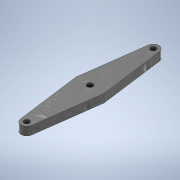
# Autodesk Inventor part: ServoXAxis
Saved by Autodesk Inventor 2022 (Build 260153000, 153)
## iProperties
Created: 2021-11-09
Part Number: ServoXAxis
Material: Generic
Document SubType Name: Modeling
Designer: Juan
Density: 1 g/cm^3
Appearance: Default
Author: Juan
Autodesk Inventor part; units mm, degrees
ref_plane "YZ Plane" through (0, 0, 0) normal (1, 0, 0) x (0, 1, 0)
ref_plane "XZ Plane" through (0, 0, 0) normal (0, 1, 0) x (-1, 0, 0)
ref_plane "XY Plane" through (0, 0, 0) normal (0, 0, 1) x (1, 0, 0)
sketch "Sketch1" plane through (0, 0, 0) normal (0, 1, 0) x (-1, 0, 0)
  circle A0 centre (0, 0) radius 2.35
  line L0 (0, 0) -> (0, -22.5)
  line L1 (0, 0) -> (0, 22.5)
  circle A1 centre (0, -22.5) radius 1
  circle A2 centre (0, 22.5) radius 1
  circle A3 centre (0, -22.5) radius 2
  circle A4 centre (0, 22.5) radius 2
  circle A5 centre (0, 0) radius 5
  line L2 (5, 0) -> (1.9827, 22.7628)
  line L3 (-5, 0) -> (-1.9827, 22.7628)
  line L4 (-5, 0) -> (-1.9827, -22.7628)
  line L5 (5, 0) -> (1.9827, -22.7628)
  circle A6 centre (0, 0) radius 1
  dimension "d0" = 4.7
  dimension "d1" = 22.5
  dimension "d2" = 22.5
  dimension "d3" = 2
  dimension "d4" = 2
  dimension "d5" = 4
  dimension "d6" = 4
  dimension "d7" = 10
  dimension "d8" = 2
  constraints: 12 end point, 7 centre point, 7 coincident, 6 point on circle, 4 tangent, 2 vertical
  measures "d0" diameter of A0
  measures "d1" distance of L0.start L0.end
  measures "d2" distance of L0.start L1.end
  measures "d3" diameter of A1
  measures "d4" diameter of A2
  measures "d5" diameter of A3
  measures "d6" diameter of A4
  measures "d7" diameter of A5
  measures "d8" diameter of A6
extrude "Extrusion1" add sketch "Sketch1" along normal blind 3 contours A0 L0 A6 L1 | A0 L1 A5 L2 L5 L0 | L1 A6 L0 A0 | A0 L0 A5 L4 L3 L1 | A5 L3 A4 L1 | L1 A4 L2 A5 | A5 L5 A3 L0 | L0 A3 L4 A5 | A4 | A3
extrude "Extrusion2" cut sketch "Sketch1" along normal blind 2.5 contours A0 L0 A6 L1 | L1 A6 L0 A0
body "Solid1"
